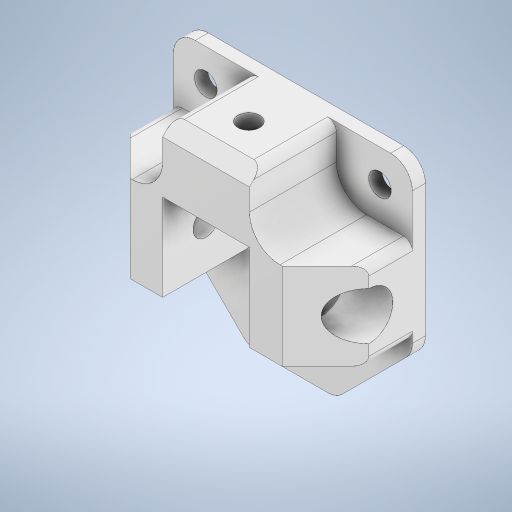
# Autodesk Inventor part: Gantry Plate
Saved by Autodesk Inventor 2023 (Build 270158000, 158)
## iProperties
Created: 2023-04-10
Part Number: Gantry Plate
Material: PC/ABS Plastic
Document SubType Name: Modeling
Designer: ethan
Density: 0.357273 g/cm^3
Appearance: Smooth - White
Author: ethan
Autodesk Inventor part; units mm, degrees
ref_plane "YZ Plane" through (0, 0, 0) normal (1, 0, 0) x (0, 1, 0)
ref_plane "XZ Plane" through (0, 0, 0) normal (0, 1, 0) x (-1, 0, 0)
ref_plane "XY Plane" through (0, 0, 0) normal (0, 0, 1) x (1, 0, 0)
sketch "Sketch1" plane through (0, 0, 0) normal (0, 1, 0) x (-1, 0, 0)
  line L0 (0, 0) -> (55, 0)
  line L1 (55, 0) -> (55, -55)
  line L2 (55, -55) -> (0, -55)
  line L3 (0, -55) -> (0, 0)
  line L4 (47.55, -7.45) -> (7.45, -7.45) construction
  line L5 (7.45, -7.45) -> (7.45, -47.55) construction
  line L6 (7.45, -47.55) -> (47.55, -47.55) construction
  line L7 (47.55, -47.55) -> (47.55, -7.45) construction
  circle A0 centre (47.55, -47.55) radius 2.6
  circle A1 centre (7.45, -47.55) radius 2.6
  circle A2 centre (27.5, -7.45) radius 3.8
  line L8 (0, -17.5) -> (17.5, 0)
  line L9 (37.5, 0) -> (55, -17.5)
  line L10 (17.5, -55) -> (37.5, -55)
  line L11 (37.5, -55) -> (37.5, -85)
  line L12 (37.5, -85) -> (17.5, -85)
  line L13 (17.5, -85) -> (17.5, -55)
  dimension "d0" = 55
  dimension "d1" = 55
  dimension "d2" = 40.1
  dimension "d3" = 40.1
  dimension "d6" = 5.2
  dimension "d7" = 5.2
  dimension "d8" = 7.45
  dimension "d9" = 7.45
  dimension "d14" = 7.6
  dimension "d55" = 20
  dimension "d56" = 10
  dimension "d84" = 20
  dimension "d85" = 30
  dimension "d86" = 17.5
  constraints: 28 end point, 6 parallel, 5 perpendicular, 5 point on line, 3 centre point, 3 horizontal, 2 coincident, 1 midpoint
  measures "d0" distance of L1.end L2.end
  measures "d1" distance of L0.end L1.end
  measures "d2" distance of L6.end L5.end
  measures "d3" distance of L5.end L4.end
  measures "d6" diameter of A0
  measures "d7" diameter of A1
  measures "d8" distance between parallel lines of L1 L7
  measures "d9" distance from line of L2 L5.end
  measures "d14" diameter of A2
  measures "d55" distance of L9.start L8.end
  measures "d56" horizontal distance of L8.end A2.centre
  measures "d84" distance of L11.end L12.end
  measures "d85" distance of L10.end L11.end
  measures "d86" distance from line of L2.end L13
extrude "Extrusion1" add sketch "Sketch1" along normal blind 3 contours L0 L9 L1 L2 L3 L8
fillet "Fillet1" radius 5 6 edges at (-55, 1.5, -55) (0, 1.5, -55) (-55, 1.5, -17.5) (-37.5, 1.5, 0) (-17.5, 1.5, 0) (0, 1.5, -17.5)
sketch "Sketch2" plane through (0, 0, 0) normal (0, -1, 0) x (1, 0, 0)
  line L0 (-17.5, -40) -> (-37.5, -40)
  line L1 (-37.5, -40) -> (-37.5, -20)
  line L2 (-37.5, -20) -> (-17.5, -20)
  line L3 (-17.5, -20) -> (-17.5, -40)
  line L4 (-5, -55) -> (-50, -55) projected
  line L5 (-17.5, -40) -> (-37.5, -40)
  line L6 (-37.5, -47) -> (-37.5, -55)
  line L7 (-37.5, -55) -> (-17.5, -55)
  line L8 (-17.5, -55) -> (-17.5, -47)
  line L9 (0, -19.5711) -> (0, -50) projected
  line L10 (-55, -50) -> (-55, -19.5711) projected
  line L11 (-10.5, -40) -> (0, -40)
  line L12 (0, -40) -> (0, -20)
  line L13 (0, -20) -> (-17.5, -20)
  line L14 (-17.5, -20) -> (-17.5, -40)
  line L15 (-44.5, -40) -> (-55, -40)
  line L16 (-55, -40) -> (-55, -20)
  line L17 (-55, -20) -> (-37.5, -20)
  line L18 (-37.5, -20) -> (-37.5, -40)
  arc A0 (-10.5, -40) -> (-17.5, -47) centre (-10.5, -47) ccw
  arc A1 (-37.5, -47) -> (-44.5, -40) centre (-44.5, -47) ccw
  point P0 (0, -40)
  point P1 (-17.5, -55)
  dimension "d68" = 20
  dimension "d69" = 20
  dimension "d70" = 55
  dimension "d71" = 17.5
  dimension "d72" = 15
  dimension "d73" = 7
  constraints: 32 end point, 9 point on line, 8 parallel, 4 horizontal, 4 perpendicular, 4 point on circle, 4 tangent, 2 centre point, 1 collinear, 1 equal radius
  measures "d68" distance of L1.end L2.end
  measures "d69" distance of L0.end L1.end
  measures "d70" distance between parallel lines of L9 L10
  measures "d71" distance between parallel lines of L8 L9
  measures "d72" distance between parallel lines of L0 L4
  measures "d73" radius of A0
extrude "Extrusion8" add sketch "Sketch2" along normal blind 20 contours L3 L13 L9 L11 A0 L8 L4 L6 A1 L15 L10 L17 L1 L0
sketch "Sketch6" plane through (-55, 0, -50) normal (-1, 0, 0) x (0, 0, 1)
  line L0 (10, -20) -> (30, -20) construction
  line L1 (10, 0) -> (30, 0) construction
  line L2 (10, -20) -> (30, 0) construction
  circle A0 centre (20, -10) radius 3
  point P0 (50, 0)
  dimension "d44" = 6
  constraints: 2 end point, 1 centre point, 1 midpoint
  measures "d44" diameter of A0
extrude "Extrusion9" cut sketch "Sketch6" against normal through all
sketch "Sketch7" plane through (-55, 0, -50) normal (-1, 0, 0) x (0, 0, 1)
  circle A0 centre (20, -10) radius 3 projected
  circle A1 centre (20, -10) radius 5.5
  point P0 (50, 0)
  dimension "d47" = 11
  constraints: 1 centre point, 1 coincident
  measures "d47" diameter of A1
extrude "Extrusion10" cut sketch "Sketch7" against normal blind 11 contours A0 | A1
sketch "Sketch8" plane through (0, 0, -50) normal (1, 0, 0) x (0, 0, -1)
  line L0 (-30, 0) -> (-30, -20) construction
  line L1 (-10, 0) -> (-30, 0) construction
  line L2 (-30, -20) -> (-10, 0) construction
  circle A0 centre (-20, -10) radius 5.5 projected
  circle A1 centre (-20, -10) radius 5.5 construction
  point P0 (-50, 0)
  constraints: 2 end point, 1 centre point, 1 coincident
extrude "Extrusion11" cut sketch "Sketch8" against normal blind 11
chamfer "Chamfer3" distance 10 angle 45 2 edges at (-55, -20, -30) (0, -20, -30)
sketch "Sketch11" plane through (-5, 3, -55) normal (0, 0, -1) x (-1, 0, 0)
  line L0 (32.5, -23) -> (12.5, -23) construction
  line L1 (12.5, -23) -> (32.1967, -3) construction
  line L2 (33.9645, -3) -> (30.4289, -3) construction
  circle A0 centre (22.3483, -13) radius 2.5
  point P0 (-5, -3)
  dimension "d74" = 5
  constraints: 2 end point, 2 midpoint, 1 centre point
  measures "d74" diameter of A0
extrude "Extrusion14" cut sketch "Sketch11" against normal blind 12.5
chamfer "Chamfer4" distance 3 angle 45 1 edges at (-27.5, -20, -55)
fillet "Fillet2" radius 2 6 edges at (-55, -5, -40) (-55, -5, -20) (0, -5, -20) (0, -5, -40) (-37.5, -8.5, -55) (-17.5, -8.5, -55)
sketch "Sketch12" plane through (0, 3, 0) normal (0, 1, 0) x (1, 0, 0)
  line L0 (-55, 50) -> (-55, 38) construction
  line L1 (0, 19.5711) -> (0, 22) construction
  line L2 (-55, 37.5) -> (0, 37.5) construction
  line L3 (0, 37.5) -> (0, 17.5) construction
  line L4 (0, 17.5) -> (-55, 17.5) construction
  line L5 (-55, 17.5) -> (-55, 37.5) construction
  circle A0 centre (-27.5, 7.45) radius 3.8 construction
  circle A1 centre (-47.55, 47.55) radius 2.6 construction
  point P0 (0, 0)
  dimension "d81" = 20
  dimension "d82" = 40.1
  dimension "d83" = 10.05
  constraints: 8 end point, 2 parallel, 2 point on line, 1 horizontal, 1 perpendicular
  measures "d81" distance of L2.end L3.end
  measures "d82" vertical distance of A0.centre A1.centre
  measures "d83" distance from line of A1.centre L2
equation "\"d1\" = d0"
equation "\"d3\" = d2"
equation "\"d8\" = -0.5 * d2 + 0.5 * d0"
equation "\"d9\" = -0.5 * d3 + 0.5 * d1"
equation "\"d86\" = -0.5 * d84 + 0.5 * d0"
equation "\"d71\" = -0.5 * d68 + 0.5 * d70"
equation "\"d83\" = -0.5 * d81 + 0.5 * d82"
body "Solid1"
